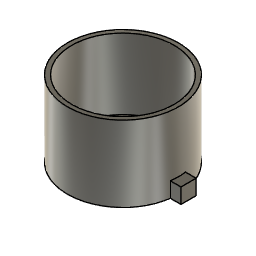
PipeCap_14x6_magnet (Autodesk Fusion 360 design; units mm, degrees)
Autodesk Fusion 360 part; units mm, degrees
note: some values were not read from the file. Chosen so that the rebuilt part matches the saved one: where a step ends.
sketch "Sketch1" plane through (0, 0, 0) normal (0, 0, 1) x (1, 0, 0)
  circle A0 centre (0, 0) radius 22
  dimension "d1" = 44
  constraint coincident A0.centre origin
  measures "d1" diameter of A0
extrude "Extrude1" add sketch "Sketch1" along normal blind 30
sketch "Sketch2" plane through (0, 0, 30) normal (0, 0, 1) x (-1, 0, 0)
  circle A0 centre (0, 0) radius 22
  circle A1 centre (0, 0) radius 20.3
  dimension "d4" = 40.6
  constraint coincident A0.centre A1.centre
  measures "d4" diameter of A1
extrude "Extrude2" cut sketch "Sketch2" against normal blind 28 contours A1
ref_plane "WorkPlane1" through (22, 0, 0) normal (1, 0, 0) x (0, 1, 0)
sketch "Sketch6" plane through (22, 0, 0) normal (1, 0, 0) x (0, 1, 0)
  line L0 (-3, 6) -> (3, 6)
  line L1 (3, 6) -> (3, 0)
  line L2 (3, 0) -> (-3, 0)
  line L3 (-3, 0) -> (-3, 6)
  line L4 (-3, 6) -> (3, 0) construction
  line L5 (3, 6) -> (-3, 0) construction
  point P0 (0, 3)
  dimension "d15" = 6
  dimension "d16" = 6
  constraint horizontal L0
  constraint perpendicular L0 L1
  constraint parallel L0 L2
  constraint parallel L1 L3
  constraint coincident L4 P0
  constraint coincident L5 P0
  measures "d15" distance of L0.start L0.end
  measures "d16" distance of L0.end L1.end
extrude "Extrude5" add sketch "Sketch6" along normal blind 4 and the other way up to near side of body 1
sketch "Sketch7" plane through (0, 0, 0) normal (0, 0, -1) x (1, 0, 0)
  line L0 (21.7945, -3) -> (26, -3)
  line L1 (26, -3) -> (26, 3)
  line L2 (26, 3) -> (21.7945, 3)
  line L3 (25.5, -2.5) -> (22.5, -2.5)
  line L4 (22.5, -2.5) -> (22.5, 2.5)
  line L5 (22.5, 2.5) -> (25.5, 2.5)
  line L6 (25.5, 2.5) -> (25.5, -2.5)
  line L7 (25.5, -2.5) -> (22.5, 2.5) construction
  line L8 (22.5, -2.5) -> (25.5, 2.5) construction
  arc A0 (21.7945, 3) -> (21.7945, -3) centre (0, 0) ccw
  point P0 (24, 0)
  dimension "d19" = 3
  dimension "d20" = 5
  constraint horizontal L3
  constraint perpendicular L3 L4
  constraint parallel L3 L5
  constraint parallel L4 L6
  constraint coincident L7 P0
  constraint coincident L8 P0
  measures "d19" distance of L4.end L5.end
  measures "d20" distance of L3.end L4.end
extrude "Extrude6" cut sketch "Sketch7" against normal blind 3 contours L3 L4 L5 L6
sketch "Sketch8" plane through (0, 0, 0) normal (0, 0, -1) x (1, 0, 0)
  line L0 (22.5, -2.5) -> (22.5, 2.5)
  line L1 (22.5, 2.5) -> (25.5, 2.5)
  line L2 (25.5, 2.5) -> (25.5, -2.5)
  line L3 (25.5, -2.5) -> (22.5, -2.5)
  arc A0 (21.7945, 3) -> (21.7945, -3) centre (0, 0) ccw
  line L4 (21.7945, -3) -> (26, -3)
  line L5 (26, -3) -> (26, 3)
  line L6 (26, 3) -> (21.7945, 3)
  circle A1 centre (0, 0) radius 8.5
  circle A2 centre (0, 0) radius 7.2
  dimension "d25" = 17
  dimension "d26" = 14.4
  constraint coincident A0.centre A1.centre
  constraint concentric A1 A2
  measures "d25" diameter of A1
  measures "d26" diameter of A2
extrude "Extrude7" add sketch "Sketch8" along normal blind 4.5 contours A1
